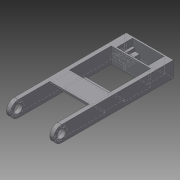
# Autodesk Inventor part: femur
Saved by Autodesk Inventor 2015 (Build 190159000, 159)
## iProperties
Created: 2016-09-30
Part Number: femur
Material: Generic
Document SubType Name: Modeling
Designer: Bardo91
Density: 1 g/cm^3
Appearance: Default
Author: Bardo91
Autodesk Inventor part; units mm, degrees
ref_plane "YZ Plane" through (0, 0, 0) normal (1, 0, 0) x (0, 1, 0)
ref_plane "XZ Plane" through (0, 0, 0) normal (0, 1, 0) x (-1, 0, 0)
ref_plane "XY Plane" through (0, 0, 0) normal (0, 0, 1) x (1, 0, 0)
sketch "Sketch1" plane through (0, 0, 0) normal (0, 0, 1) x (1, 0, 0)
  line L0 (0, 0) -> (-25, 0)
  line L1 (-25, 0) -> (-25, 150)
  line L2 (-25, 150) -> (-30, 150)
  line L3 (-30, 150) -> (-30, 0)
  line L4 (-30, 0) -> (-25, 0)
  line L5 (0, 0) -> (25, 0)
  line L6 (25, 0) -> (25, 150)
  line L7 (25, 150) -> (30, 150)
  line L8 (30, 150) -> (30, 0)
  line L9 (30, 0) -> (25, 0)
  dimension "d0" = 25
  dimension "d1" = 150
  dimension "d2" = 5
  dimension "d3" = 25
  dimension "d4" = 5
  constraints: 20 end point, 6 perpendicular, 5 point on line, 1 horizontal, 1 parallel
  measures "d0" distance of L0.start L0.end
  measures "d1" distance of L0.end L1.end
  measures "d2" distance of L1.end L2.end
  measures "d3" distance of L0.start L5.end
  measures "d4" distance of L6.end L7.end
extrude "Extrusion1" add sketch "Sketch1" along normal blind 20
fillet "Fillet1" radius 10 4 edges at (27.5, 0, 20) (-27.5, 0, 20) (-27.5, 0, 0) (27.5, 0, 0)
sketch "Sketch2" plane through (30, 10, 0) normal (1, 0, 0) x (0, 0, -1)
  arc A0 (-20, 0) -> (0, 0) centre (-10, 0) ccw projected
  line L0 (-10, 0) -> (-20, 0)
  circle A1 centre (-10, 0) radius 5.5
  line L1 (-10, 0) -> (-17.5, 0)
  circle A2 centre (-17.5, 0) radius 0.75
  circle A3 centre (-15.3033, -5.3033) radius 0.75
  circle A4 centre (-10, -7.5) radius 0.75
  circle A5 centre (-4.6967, -5.3033) radius 0.75
  circle A6 centre (-2.5, 0) radius 0.75
  circle A7 centre (-4.6967, 5.3033) radius 0.75
  circle A8 centre (-10, 7.5) radius 0.75
  circle A9 centre (-15.3033, 5.3033) radius 0.75
  point P0 (0, -10)
  dimension "d8" = 11
  dimension "d11" = 7.5
  dimension "d12" = 1.5
  dimension "d15" = 360
  constraints: 9 centre point, 4 end point, 2 coincident, 1 point on circle, 1 point on line, 17 other
  measures "d8" diameter of A1
  measures "d11" distance of L1.start L1.end
  measures "d12" diameter of A2
extrude "Extrusion2" cut sketch "Sketch2" against normal through all
sketch "Sketch3" plane through (30, 10, 0) normal (1, 0, 0) x (0, 0, -1)
  line L0 (0, 0) -> (-20, 0)
  line L1 (-20, 140) -> (-20, 0) projected
  line L2 (-20, 0) -> (-20, 40)
  line L3 (-20, 40) -> (-17.5, 40)
  line L4 (-17.5, 40) -> (-17.5, 65)
  line L5 (-17.5, 65) -> (-20, 65)
  line L6 (-20, 40) -> (-20, 65)
  line L7 (0, 0) -> (0, 60)
  line L8 (0, 60) -> (-2.5, 60)
  line L9 (-2.5, 60) -> (-2.5, 85)
  line L10 (-2.5, 85) -> (0, 85)
  line L11 (0, 85) -> (0, 60)
  line L12 (0, 0) -> (0, 140) projected
  point P0 (0, -10)
  point P1 (-20, 130)
  point P2 (0, 130)
  dimension "d17" = 40
  dimension "d18" = 2.5
  dimension "d19" = 25
  dimension "d20" = 60
  dimension "d21" = 2.5
  dimension "d22" = 25
  constraints: 22 end point, 5 perpendicular, 3 point on line, 2 collinear, 1 horizontal, 1 parallel
  measures "d17" distance of L0.end L2.end
  measures "d18" distance of L2.end L3.end
  measures "d19" distance of L3.end L4.end
  measures "d20" distance of L0.start L7.end
  measures "d21" distance of L7.end L8.end
  measures "d22" distance of L8.end L9.end
extrude "Extrusion3" add sketch "Sketch3" against normal up to surface (60 mm away)
sketch "Sketch4" plane through (-30, 150, 0) normal (0, 1, 0) x (1, 0, 0)
  line L0 (5, 0) -> (19, 0)
  line L1 (55, 0) -> (5, 0) projected
  line L2 (19, 0) -> (19, -7)
  line L3 (19, -7) -> (13, -7)
  line L4 (13, -7) -> (13, -11)
  line L5 (13, -11) -> (10, -11)
  line L6 (10, -11) -> (10, -20)
  line L7 (55, -20) -> (5, -20) projected
  line L8 (10, -20) -> (5, -20)
  line L9 (5, -17.5) -> (5, -20) projected
  line L10 (5, -20) -> (5, 0)
  point P0 (30, 0)
  dimension "d25" = 14
  dimension "d26" = 7
  dimension "d27" = 6
  dimension "d28" = 4
  dimension "d29" = 3
  constraints: 16 end point, 7 perpendicular, 2 point on line
  measures "d25" distance of L0.start L0.end
  measures "d26" distance of L0.end L2.end
  measures "d27" distance of L2.end L3.end
  measures "d28" distance of L3.end L4.end
  measures "d29" distance of L4.end L5.end
extrude "Extrusion4" add sketch "Sketch4" against normal blind 20
sketch "Sketch5" plane through (-25, 10, 10) normal (1, 0, 0) x (0, 0, -1)
  line L0 (-10, 120) -> (-10, 118)
  line L1 (-10, 140) -> (-10, 0) projected
  line L2 (-10, 118) -> (10, 118)
  line L3 (10, 118) -> (10, 120)
  line L4 (10, 140) -> (10, 0) projected
  line L5 (-1, 120) -> (-10, 120) projected
  line L6 (-10, 120) -> (10, 120)
  point P0 (10, -10)
  dimension "d32" = 2
  constraints: 8 end point, 3 perpendicular, 2 point on line
  measures "d32" distance of L0.start L0.end
extrude "Extrusion5" add sketch "Sketch5" along normal up to surface (55 mm away)
sketch "Sketch6" plane through (-20, 130, 20) normal (0, 1, 0) x (1, 0, 0)
  line L0 (45, 20) -> (40, 20)
  line L1 (45, 20) -> (-5, 20) projected
  line L2 (40, 20) -> (40, 0)
  line L3 (40, 0) -> (45, 0)
  line L4 (45, 0) -> (-5, 0) projected
  line L5 (45, 0) -> (40, 0)
  line L6 (45, 0) -> (45, 20)
  point P0 (20, 20)
  dimension "d35" = 5
  constraints: 10 end point, 2 collinear, 2 perpendicular, 1 point on line
  measures "d35" distance of L0.start L0.end
extrude "Extrusion6" add sketch "Sketch6" along normal up to surface (20 mm away)
sketch "Sketch7" plane through (30, 150, 20) normal (0, 1, 0) x (1, 0, 0)
  line L0 (0, 0) -> (-59.9569, 0)
  line L1 (-59.9569, 0) -> (-59.9569, 20)
  line L2 (-59.9569, 20) -> (0, 20)
  line L3 (0, 20) -> (0, 0)
  point P0 (-30, 20)
  constraints: 8 end point, 3 perpendicular, 1 horizontal
extrude "Extrusion7" add sketch "Sketch7" along normal blind 2
sketch "Sketch8" plane through (-30, 150, 0) normal (-1, 0, 0) x (0, 0, 1)
  line L0 (7, 0) -> (7, -20)
  line L1 (7, 0) -> (7, -20) projected
  line L2 (7, -10) -> (5, -10)
  line L3 (5, -10) -> (5, -15)
  line L4 (5, -15) -> (2.5, -15)
  circle A0 centre (2.5, -15) radius 3
  line L5 (5, -10) -> (5, -5)
  line L6 (5, -5) -> (2.5, -5)
  circle A1 centre (2.5, -5) radius 3
  point P0 (0, -150)
  dimension "d40" = 2
  dimension "d41" = 5
  dimension "d42" = 2.5
  dimension "d43" = 6
  dimension "d44" = 5
  dimension "d45" = 2.5
  dimension "d46" = 6
  constraints: 12 end point, 2 centre point, 2 coincident, 2 horizontal, 2 perpendicular, 1 collinear, 1 midpoint, 1 vertical
  measures "d40" distance of L2.start L2.end
  measures "d41" distance of L2.end L3.end
  measures "d42" distance of L3.end L4.end
  measures "d43" diameter of A0
  measures "d44" distance of L2.end L5.end
  measures "d45" distance of L5.end L6.end
  measures "d46" diameter of A1
extrude "Extrusion8" cut sketch "Sketch8" against normal up to surface (19 mm away)
equation "\"d9\" = d8"
body "Solid1"
